Autodesk Fusion 360 part; units mm, degrees
(part 4 of 4)
sketch "profiles" plane through (0, 0, 0) normal (0, 0, 1) x (1, 0, 0)
  arc A0 (18.525, 0) -> (19.325, 25.4) centre (-384.3, 25.4) ccw
  line L0 (19.325, 25.4) -> (19.325, 114.25)
  line L1 (19.325, 114.25) -> (22.5, 114.25)
  line L2 (22.5, 114.25) -> (22.5, 0) construction
  line L3 (22.5, 0) -> (18.525, 0)
  line L4 (22.5, 0) -> (26.475, 0)
  arc A1 (25.675, 25.4) -> (26.475, 0) centre (429.3, 25.4) ccw
  line L5 (25.675, 25.4) -> (25.675, 114.25)
  line L6 (25.675, 114.25) -> (22.5, 114.25)
  line L7 (0, 0) -> (315, 0)
  line L8 (67.5, 0) -> (67.5, 114.25) construction
  line L9 (202.5, 0) -> (202.5, 106) construction
  line L10 (292.5, 144.5) -> (292.5, 0) construction
  line L11 (67.5, 114.25) -> (61.15, 114.25)
  line L12 (61.15, 114.25) -> (61.15, 27)
  line L13 (63.5, 0) -> (67.5, 0)
  arc A2 (63.5, 0) -> (61.15, 27) centre (-92.7814, 0) ccw
  line L14 (67.5, 114.25) -> (73.85, 114.25)
  line L15 (73.85, 114.25) -> (73.85, 27)
  arc A3 (73.85, 27) -> (71.5, 0) centre (227.7814, 0) ccw
  line L16 (71.5, 0) -> (67.5, 0)
  line L17 (112.5, 114.25) -> (122.025, 114.25)
  line L18 (122.025, 114.25) -> (122.025, 26.5)
  arc A4 (122.025, 26.5) -> (116.475, 0) centre (182.5158, 0) ccw
  line L19 (116.475, 0) -> (112.5, 0)
  line L20 (102.975, 114.25) -> (102.975, 26.5)
  arc A5 (108.525, 0) -> (102.975, 26.5) centre (42.4842, 0) ccw
  line L21 (108.525, 0) -> (112.5, 0)
  line L22 (112.5, 114.25) -> (102.975, 114.25)
  line L23 (112.5, 0) -> (112.5, 114.25) construction
  line L24 (157.5, 63.25) -> (176.55, 63.25)
  line L25 (176.55, 63.25) -> (176.55, 33.5)
  arc A6 (176.55, 33.5) -> (161.475, 0) centre (206.2347, 0) ccw
  line L26 (161.475, 0) -> (157.5, 0)
  line L27 (138.45, 63.25) -> (138.45, 33.5)
  arc A7 (153.525, 0) -> (138.45, 33.5) centre (108.7653, 0) ccw
  line L28 (153.525, 0) -> (157.5, 0)
  line L29 (157.5, 63.25) -> (138.45, 63.25)
  line L30 (157.5, 0) -> (157.5, 63.25) construction
  line L31 (247.5, 168.5) -> (260.2, 168.5)
  line L32 (260.2, 168.5) -> (260.2, 11.5)
  arc A8 (260.2, 11.5) -> (251, 0) centre (262.7875, 0) ccw
  line L33 (251, 0) -> (247.5, 0)
  line L34 (234.8, 168.5) -> (234.8, 11.5)
  arc A9 (244, 0) -> (234.8, 11.5) centre (232.2125, 0) ccw
  line L35 (244, 0) -> (247.5, 0)
  line L36 (247.5, 168.5) -> (234.8, 168.5)
  line L37 (247.5, 0) -> (247.5, 168.5) construction
  line L38 (202.5, 106) -> (197.7375, 106)
  line L39 (197.7375, 106) -> (197.7375, 0)
  line L40 (197.7375, 0) -> (202.5, 0)
  line L41 (202.5, 106) -> (207.2625, 106)
  line L42 (207.2625, 106) -> (207.2625, 0)
  line L43 (207.2625, 0) -> (202.5, 0)
  line L44 (292.5, 144.5) -> (288.5, 144.5)
  line L45 (288.5, 144.5) -> (288.5, 31)
  line L46 (288.5, 31) -> (281.5, 0) construction
  line L47 (292.5, 0) -> (281.5, 0)
  line L48 (292.5, 144.5) -> (296.5, 144.5)
  line L49 (296.5, 144.5) -> (296.5, 31)
  line L50 (296.5, 31) -> (303.5, 0) construction
  line L51 (292.5, 0) -> (303.5, 0)
  arc A10 (288.5, 31) -> (281.5, 0) centre (353.6429, 0) ccw
  arc A11 (303.5, 0) -> (296.5, 31) centre (231.3571, 0) ccw
  line L52 (288.5, 31) -> (296.5, 31)
  line L53 (0, 0) -> (0, 187)
  line L54 (0, 187) -> (315, 187)
  line L55 (315, 187) -> (315, 0)
  line L56 (0, 132.75) -> (216.3, 132.75)
  line L57 (216.3, 132.75) -> (216.3, 187)
  line L58 (216.3, 132.75) -> (216.3, 0) construction
  line L59 (0, 66.375) -> (315, 66.375) construction
  circle A12 centre (43.4125, 66.375) radius 5
  circle A13 centre (274.35, 66.375) radius 5
  line L60 (25.675, 114.25) -> (43.4125, 66.375) construction
  line L61 (61.15, 114.25) -> (43.4125, 66.375) construction
  line L62 (288.5, 144.5) -> (274.35, 66.375) construction
  line L63 (274.35, 66.375) -> (260.2, 144.5) construction
  line L64 (288.5, 144.5) -> (260.2, 144.5) construction
  circle A14 centre (22.5, 102.25) radius 3.175
  circle A15 centre (22.5, 92.25) radius 3.175
  circle A16 centre (22.5, 82.25) radius 3.175
  circle A17 centre (67.5, 102.25) radius 3.175
  circle A18 centre (112.5, 102.25) radius 3.175
  circle A19 centre (67.5, 92.25) radius 3.175
  circle A20 centre (112.5, 92.25) radius 3.175
  circle A21 centre (67.5, 82.25) radius 3.175
  circle A22 centre (112.5, 82.25) radius 3.175
  circle A23 centre (157.5, 51.25) radius 3.175
  circle A24 centre (157.5, 41.25) radius 3.175
  circle A25 centre (157.5, 31.25) radius 3.175
  circle A26 centre (202.5, 94) radius 3.175
  circle A27 centre (202.5, 84) radius 3.175
  circle A28 centre (202.5, 74) radius 3.175
  circle A29 centre (247.5, 156.5) radius 3.175
  circle A30 centre (247.5, 146.5) radius 3.175
  circle A31 centre (247.5, 136.5) radius 3.175
  circle A32 centre (292.5, 132.5) radius 3.175
  circle A33 centre (292.5, 122.5) radius 3.175
  circle A34 centre (292.5, 112.5) radius 3.175
  circle A35 centre (157.5, 98) radius 5
  line L65 (157.5, 63.25) -> (157.5, 98) construction
  line L66 (157.5, 98) -> (157.5, 132.75) construction
  circle A36 centre (292.5, 102.5) radius 3.175
  circle A37 centre (292.5, 92.5) radius 3.175
  circle A38 centre (292.5, 82.5) radius 3.175
  circle A39 centre (292.5, 72.5) radius 3.175
  circle A40 centre (292.5, 62.5) radius 3.175
  circle A41 centre (292.5, 52.5) radius 3.175
  circle A42 centre (292.5, 42.5) radius 3.175
  point P0 (216.3, 66.375)
  dimension "d1" = 7.95
  dimension "d2" = 6.35
  dimension "d3" = 25.4
  dimension "d4" = 22.5
  dimension "d5" = 114.25
  dimension "d6" = 12.7
  dimension "d7" = 114.25
  dimension "d8" = 45
  dimension "d9" = 8
  dimension "d10" = 27
  dimension "d11" = 26.5
  dimension "d12" = 19.05
  dimension "d13" = 114.25
  dimension "d14" = 45
  dimension "d15" = 7.95
  dimension "d16" = 7.95
  dimension "d17" = 38.1
  dimension "d18" = 63.25
  dimension "d19" = 45
  dimension "d20" = 33.5
  dimension "d21" = 7
  dimension "d22" = 25.4
  dimension "d23" = 168.5
  dimension "d24" = 45
  dimension "d25" = 45
  dimension "d26" = 11.5
  dimension "d27" = 9.525
  dimension "d28" = 106
  dimension "d29" = 45
  dimension "d30" = 113.5
  dimension "d31" = 8
  dimension "d32" = 22
  dimension "d33" = 31
  dimension "d34" = 22.5
  dimension "d35" = 315
  dimension "d38" = 18.5
  dimension "d39" = 18.5
  dimension "d40" = 18.5
  dimension "d41" = 18.5
  dimension "d42" = 132.75
  dimension "d43" = 187
  dimension "d44" = 10
  dimension "d47" = 6.35
  dimension "d48" = 12
  dimension "d51" = 45
  dimension "d52" = -10
  dimension "d56" = 0
  dimension "d57" = -10
  dimension "d60" = 0
  dimension "d61" = -10
  dimension "d65" = 0
  dimension "d66" = -10
  dimension "d70" = 0
  dimension "d71" = -10
  dimension "d73" = 12
  dimension "d74" = 12
  dimension "d75" = 12
  dimension "d76" = 12
  dimension "d88" = 54.25
  dimension "d89" = 216.3
  constraint vertical L2
  constraint horizontal L1
  constraint vertical L0
  constraint tangent A0 L0
  constraint horizontal L3
  constraint symmetric A0.start L2 L4.end
  constraint symmetric A0.end L2 A1.start
  constraint symmetric A0 L2 A1
  constraint symmetric L0.end L2 L5.end
  constraint coincident L7.start L53.start
  constraint horizontal L7
  constraint coincident A0.start L7
  constraint vertical L8
  constraint coincident L7 L8.start
  constraint coincident L7 L9.start
  constraint coincident L7 L10.end
  constraint vertical L10
  constraint coincident L7 L13.start
  constraint vertical L12
  constraint horizontal L11
  constraint symmetric L8 L11.end L14.end
  constraint symmetric L8 L12.end L15.end
  constraint symmetric L8 L13.start A3.end
  constraint symmetric L8 A2 A3
  constraint coincident L7 A3.end
  constraint vertical L23
  constraint vertical L20
  constraint horizontal L22
  constraint symmetric L17.end L20.start L23
  constraint symmetric L18.end L20.end L23
  constraint symmetric A5.start A4.end L23
  constraint symmetric A4 A5 L23
  constraint vertical L30
  constraint vertical L27
  constraint horizontal L29
  constraint symmetric L24.end L27.start L30
  constraint symmetric L25.end L27.end L30
  constraint symmetric A7.start A6.end L30
  constraint symmetric A6 A7 L30
  constraint vertical L37
  constraint vertical L34
  constraint horizontal L36
  constraint symmetric L33.end L35.end L37
  constraint symmetric L31.end L34.start L37
  constraint symmetric L32.end L34.end L37
  constraint symmetric A9.start A8.end L37
  constraint symmetric A8 A9 L37
  constraint coincident L7 A2.centre
  constraint coincident L7 A5.centre
  constraint coincident L7 A5.start
  constraint coincident L7 L19.end
  constraint coincident L7 A6.end
  constraint coincident L7 L26.end
  constraint coincident L7 A7.centre
  constraint coincident L7 A9.centre
  constraint coincident L7 A9.start
  constraint coincident L7 L33.end
  constraint coincident L7 L39.end
  constraint vertical L39
  constraint horizontal L38
  constraint symmetric L9 L38.end L41.end
  constraint symmetric L9 L39.end L42.end
  constraint coincident L7 L42.end
  constraint coincident L7 L46.end
  constraint vertical L45
  constraint horizontal L44
  constraint symmetric L10 L44.end L48.end
  constraint symmetric L10 L45.end L49.end
  constraint symmetric L10 L46.end L50.end
  constraint symmetric L10 A10 A11
  constraint coincident L7 A10.centre
  constraint vertical L55
  constraint horizontal L54
  constraint vertical L53
  constraint coincident L53 L56.start
  constraint coincident L54 L57.end
  constraint horizontal L56
  constraint vertical L57
  constraint coincident L7 L58.end
  constraint vertical L58
  constraint coincident L53 L59.start
  constraint coincident L55 L59.end
  constraint horizontal L59
  constraint midpoint L58 P0
  constraint coincident L59 P0
  constraint coincident L59 A12.centre
  constraint coincident L59 A13.centre
  constraint equal A12 A13
  constraint coincident A12.centre L60.end
  constraint coincident A13.centre L62.end
  constraint coincident L32 L63.end
  constraint horizontal L64
  constraint equal L62 L63
  constraint equal L60 L61
  constraint coincident L2 A14.centre
  constraint coincident L30 A23.centre
  constraint equal A14 A23
  constraint equal A14 A26
  constraint equal A14 A29
  constraint equal A14 A32
  constraint coincident L9 A26.centre
  constraint coincident L37 A29.centre
  constraint coincident L10 A32.centre
  constraint coincident A35.centre L65.end
  constraint perpendicular L59 L65
  constraint equal A12 A35
  constraint coincident L56 L66.end
  constraint vertical L66
  constraint equal L65 L66
  measures "d1" distance of A0.start L4.end
  measures "d2" distance of L0.end L5.end
  measures "d3" vertical distance of A0.start A0.end
  measures "d4" distance of L7.start L2.end
  measures "d5" vertical distance of A0.start L0.end
  measures "d6" distance of L11.end L14.end
  measures "d7" distance of L7 L11.end
  measures "d8" distance of L2.end L8.start
  measures "d9" distance of L13.start A3.end
  measures "d10" vertical distance of L12.end L13.start
  measures "d11" vertical distance of A5.start L20.end
  measures "d12" distance of L17.end L20.start
  measures "d13" vertical distance of A5.start L20.start
  measures "d14" distance of L8.start L19.end
  measures "d15" distance of A5.start A4.end
  measures "d16" distance of A7.start A6.end
  measures "d17" distance of L24.end L27.start
  measures "d18" vertical distance of A7.start L27.start
  measures "d19" distance of L19.end L26.end
  measures "d20" vertical distance of A7.start L27.end
  measures "d21" distance of A9.start A8.end
  measures "d22" distance of L31.end L34.start
  measures "d23" vertical distance of A9.start L34.start
  measures "d24" distance of L26.end L9.start
  measures "d25" distance of L33.end L9.start
  measures "d26" vertical distance of A9.start L34.end
  measures "d27" distance of L38.end L41.end
  measures "d28" distance of L38.end L39.end
  measures "d29" distance of L33.end L10.end
  measures "d30" distance of L44.end L45.end
  measures "d31" distance of L44.end L48.end
  measures "d32" distance of L46.end L50.end
  measures "d33" vertical distance of L45.end L46.end
  measures "d34" distance of L7.end L10.end
  measures "d35" distance of L53.end L54.end
  measures "d38" horizontal distance of L48.end L54.end
  measures "d39" horizontal distance of L34.start L57.end
  measures "d40" vertical distance of L34.start L57.end
  measures "d41" vertical distance of L0.end L56.start
  measures "d42" distance of L7.start L56.start
  measures "d43" distance of L7.start L53.end
  measures "d44" diameter of A12
  measures "d47" diameter of A14
  measures "d48" vertical distance of L0.end A14.centre
  measures "d73" vertical distance of L27.start A23.centre
  measures "d74" distance of L9.end A26.centre
  measures "d75" vertical distance of L34.start A29.centre
  measures "d76" distance of L10.start A32.centre
  measures "d88" distance of L53.end L56.start
  measures "d89" distance of L53.end L57.end
extrude "Extrude1" add sketch "profiles" against normal blind 12.7 contours A0 L0 L1 A1 L5 L6 L7 L11 L12 A2 L14 L15 A3 L17 L18 A4 L20 A5 L22 L24 L25 A6 L27 A7 L29 L31 L32 A8 L34 A9 L36 L38 L39 L41 L42 L44 L45 L48 L49 A10 A11 L53 L54 L55 L56 L57 | A0 L0 L3 L4 A1 L5 L7 A16 | L0 L5 A15 A16 | A16 | L0 L5 A14 A15 | A15 | L7 L11 L12 L13 A2 L14 L15 A3 L16 | L0 L1 L5 L6 A14 | A14 | L7 L17 L18 A4 L19 L20 A5 L21 L22 | L44 L45 L48 L49 L52 | L7 L24 L25 A6 L26 L27 A7 L28 L29 | L7 L31 L32 A8 L33 L34 A9 L35 L36 | L7 L38 L39 L40 L41 L42 L43 | A12 | A13 | A17 | A18 | A19 | A20 | A21 | A22 | A23 | A24 | A25 | A26 | A27 | A28 | A29 | A30 | A31 | A32 | A33 | A34 | A35 | A36 | A37 | A38 | A39 | A40 | A41 | A42
extrude "Extrude2" cut sketch "profiles" against normal blind 2 contours A0 L0 L3 L4 A1 L5 L7 A16 | L0 L5 A15 A16 | L0 L5 A14 A15 | L7 L11 L12 L13 A2 L14 L15 A3 L16 | L0 L1 L5 L6 A14 | L7 L17 L18 A4 L19 L20 A5 L21 L22 | L44 L45 L48 L49 L52 | L7 L24 L25 A6 L26 L27 A7 L28 L29 | L7 L31 L32 A8 L33 L34 A9 L35 L36 | L7 L38 L39 L40 L41 L42 L43
extrude "Extrude3" cut sketch "profiles" along normal blind -4 and the other way blind -100 from surface at -2 contours A16 | A15 | A14 | A17 | A18 | A19 | A20 | A21 | A22 | A23 | A24 | A25 | A26 | A27 | A28 | A29 | A30 | A31 | A32 | A33 | A34 | A36 | A37 | A38 | A39 | A40 | A41 | A42
extrude "Extrude4" cut sketch "profiles" against normal up to surface (6.7 mm away) contours A12 | A13 | A35
chamfer "Chamfer1" distance 4 angle 45 5 edges at (265.65, 187, 0) (216.3, 159.875, 0) (315, 93.5, 0) (108.15, 132.75, 0) (0, 66.375, 0)
equation "d2 = 1/4\""
equation "d3 = 1\""
equation "d4 = d8 / 2"
equation "d6 = 1/2\""
equation "d12 = 3/4\""
equation "d14 = d8"
equation "d19 = d8"
equation "d22 = 1\""
equation "d24 = d8"
equation "d25 = d8"
equation "d27 = 3/8\""
equation "d29 = d8"
equation "d34 = d4"
equation "d39 = d38"
equation "d40 = d39"
equation "d41 = d39"
equation "d45 = d8"
equation "d47 = 1/4\""
equation "d73 = d48"
equation "d74 = d48"
equation "d75 = d48"
equation "d76 = d48"
equation "d77 = -1/2\""
